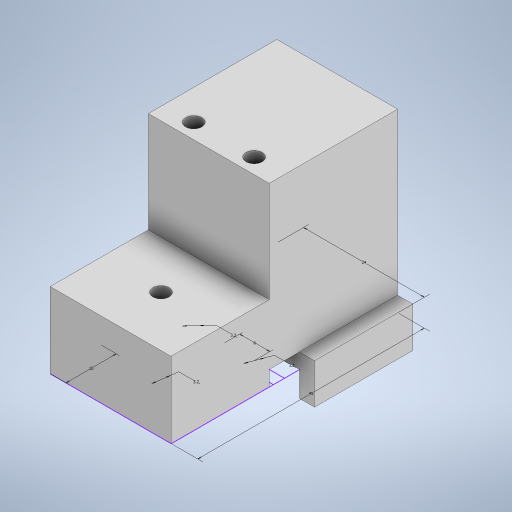
# Autodesk Inventor part: spoutstandsupport
Saved by Autodesk Inventor 2023 (Build 270158000, 158)
## iProperties
Created: 2025-10-04
Part Number: spoutstandsupport
Material: Generic
Document SubType Name: Modeling
Designer: ptato_qo49uko
Density: 1 g/cm^3
Appearance: Default
Author: ptato_qo49uko
Autodesk Inventor part; units mm, degrees
ref_plane "YZ Plane" through (0, 0, 0) normal (1, 0, 0) x (0, 1, 0)
ref_plane "XZ Plane" through (0, 0, 0) normal (0, 1, 0) x (-1, 0, 0)
ref_plane "XY Plane" through (0, 0, 0) normal (0, 0, 1) x (1, 0, 0)
sketch "Sketch2" plane through (0, 0, 0) normal (0, 1, 0) x (-1, 0, 0)
  line L0 (12, 22.5) -> (-12, 22.5)
  line L1 (-12, 22.5) -> (-12, -22.5)
  line L2 (-12, -22.5) -> (12, -22.5)
  line L3 (12, -22.5) -> (12, 22.5)
  line L4 (12, 22.5) -> (12, 12.5)
  line L5 (12, 12.5) -> (0, 12.5)
  circle A0 centre (0, 12.5) radius 1.6
  line L6 (0, 12.5) -> (0, 0)
  line L7 (0, 0) -> (-6, 0)
  line L8 (-6, 0) -> (6, 0)
  circle A1 centre (-6, 0) radius 1.6
  circle A2 centre (6, 0) radius 1.6
  line L9 (-12, 22.5) -> (12, 22.5)
  line L10 (12, 22.5) -> (12, 0)
  line L11 (12, 0) -> (-12, 0)
  line L12 (-12, 0) -> (-12, 22.5)
  line L13 (-12, 22.5) -> (12, 22.5)
  line L14 (12, 22.5) -> (12, 2.2056)
  line L15 (12, 2.2056) -> (-12, 2.2056)
  line L16 (-12, 2.2056) -> (-12, 22.5)
  dimension "d0" = 24
  dimension "d1" = 45
  dimension "d2" = 10
  dimension "d3" = 3.2
  dimension "d6" = 6
  dimension "d7" = 3.2
  dimension "d8" = 3.2
  constraints: 34 end point, 6 parallel, 5 perpendicular, 3 centre point, 3 coincident, 3 horizontal, 3 point on line, 1 midpoint, 1 vertical
  measures "d0" distance of L2.end L1.end
  measures "d1" distance of L1.end L0.end
  measures "d2" distance of L0.start L4.end
  measures "d3" diameter of A0
  measures "d6" distance of L6.end L7.end
  measures "d7" diameter of A1
  measures "d8" diameter of A2
extrude "Extrusion1" add sketch "Sketch2" along normal blind 35 contours L3 L5 A0 L6 L15 L1 L0 | L3 L15 L6 A0 L5 | L15 L6 L7 A1 L11 L1 | L3 L11 A2 L8 L6 L15 | L11 A1 L7 L8 A2 L3 L2 L1 | L11 L7 A1 | A1 L7 L11 | L11 L8 A2 | A2 L8 L11
sketch "Sketch3" plane through (0, 0, 0) normal (0, -1, 0) x (1, 0, 0)
  line L0 (12, 22.5) -> (12, -22.5) projected
  line L1 (-12, -22.5) -> (-12, 22.5) projected
  line L2 (12, 3) -> (-12, 3)
  line L3 (-12, 3) -> (-12, -3)
  line L4 (-12, -3) -> (12, -3)
  line L5 (12, -3) -> (12, 3)
  point P0 (0, 0)
  dimension "d9" = 6
  constraints: 8 end point, 2 parallel, 2 point on line, 1 horizontal, 1 perpendicular
  measures "d9" distance of L3.end L2.end
extrude "Extrusion2" cut sketch "Sketch3" against normal blind 3
hole "Hole1" at (-6, 0, 0) at (6, 0, 0) direction (0, 1, 0) diameter 3.2 depth 44.75 countersink diameter 4 countersink angle 90
sketch "Sketch4" plane through (0, 35, 0) normal (0, 1, 0) x (1, 0, 0)
  line L0 (12, -3) -> (12, 3) projected
  line L1 (-12, -22.5) -> (12, -22.5)
  line L2 (12, -22.5) -> (12, -3)
  line L3 (12, -3) -> (-12, -3)
  line L4 (-12, -3) -> (-12, -22.5)
  point P0 (0, 0)
  constraints: 8 end point, 2 parallel, 1 horizontal, 1 perpendicular
extrude "Extrusion3" cut sketch "Sketch4" against normal blind 20
sketch "Sketch5" plane through (12, 0, -22.5) normal (1, 0, 0) x (0, 0, -1)
  line L0 (-45, 0) -> (-25.5, 0) projected
  line L1 (-45, 0) -> (-45, 15) projected
  line L2 (-25.5, 0) -> (-45, 0)
  line L3 (-45, 0) -> (-45, 3)
  line L4 (-45, 3) -> (-25.5, 3)
  line L5 (-25.5, 3) -> (-25.5, 0)
  point P0 (-22.5, 0)
  dimension "d21" = 3
  constraints: 8 end point, 2 parallel, 1 horizontal, 1 perpendicular, 1 point on line
  measures "d21" distance of L2.end L3.end
extrude "Extrusion4" add sketch "Sketch5" along normal blind 3
sketch "Sketch6" plane through (0, 0, 0) normal (0, -1, 0) x (1, 0, 0)
  line L0 (-12, 3) -> (15, 3) projected
  line L1 (12, 22.5) -> (12, 3) projected
  line L2 (15, 3) -> (12, 3)
  line L3 (12, 3) -> (12, 22.5)
  line L4 (12, 22.5) -> (15, 22.5)
  line L5 (15, 22.5) -> (15, 3)
  point P0 (0, 0)
  constraints: 8 end point, 2 parallel, 1 horizontal, 1 perpendicular
extrude "Extrusion5" add sketch "Sketch6" along normal blind 5
sketch "Sketch7" plane through (-12, 0, 3) normal (0, 0, -1) x (-1, 0, 0)
  line L0 (-24, 0) -> (-24, -5) projected
  line L1 (-27, 3) -> (-27, -5) projected
  line L2 (-24, -5) -> (-27, -5)
  line L3 (-27, -5) -> (-27, 3)
  line L4 (-27, 3) -> (-24, 3)
  line L5 (-24, 3) -> (-24, -5)
  point P0 (-12, 0)
  constraints: 8 end point, 2 parallel, 1 horizontal, 1 perpendicular
extrude "Extrusion6" add sketch "Sketch7" along normal blind 25.5
sketch "Sketch8" plane through (-12, 15, 22.5) normal (0, 0, 1) x (1, 0, 0)
  line L0 (27, -12) -> (27, -20) projected
  line L1 (24, -12) -> (24, -15) projected
  line L2 (27, -20) -> (24, -20)
  line L3 (24, -20) -> (24, -12)
  line L4 (24, -12) -> (27, -12)
  line L5 (27, -12) -> (27, -20)
  point P0 (12, -15)
  constraints: 8 end point, 2 parallel, 1 horizontal, 1 perpendicular
extrude "Extrusion7" cut sketch "Sketch8" against normal blind 25.5
body "Solid1"
